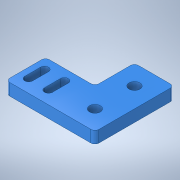
# Autodesk Inventor part: Belt_Clamp
Saved by Autodesk Inventor 2021 (Build 250183000, 183)
## iProperties
Created: 2021-02-02
Part Number: Belt_Clamp
Material: Generic
Document SubType Name: Modeling
Designer: Jorian Brusind
Density: 1 g/cm^3
Appearance: Cyan
Author: Jorian Brusind
Autodesk Inventor part; units mm, degrees
ref_plane "YZ Plane" through (0, 0, 0) normal (1, 0, 0) x (0, 1, 0)
ref_plane "XZ Plane" through (0, 0, 0) normal (0, 1, 0) x (-1, 0, 0)
ref_plane "XY Plane" through (0, 0, 0) normal (0, 0, 1) x (1, 0, 0)
sketch "Sketch1" plane through (0, 0, 0) normal (0, 1, 0) x (-1, 0, 0)
  line L0 (0, 0) -> (45, 0)
  line L1 (45, 0) -> (45, -40)
  line L2 (45, -40) -> (0, -40)
  line L3 (0, -40) -> (0, 0)
  line L4 (45, 0) -> (45, -20)
  line L5 (45, -20) -> (20, -20)
  line L6 (20, -20) -> (20, -40)
  dimension "d0" = 45
  dimension "d1" = 40
  dimension "d13" = 20
  dimension "d14" = 25
  constraints: 14 end point, 3 perpendicular, 2 parallel, 1 horizontal, 1 midpoint, 1 point on line
  measures "d0" distance of L1.end L2.end
  measures "d1" distance of L0.end L1.end
  measures "d13" distance of L0.end L4.end
  measures "d14" distance of L4.end L5.end
extrude "Extrusion3" add sketch "Sketch1" along normal blind 6 contours L0 L1 L5 L6 L2 L3
sketch "Sketch4" plane through (0, 6, 0) normal (0, 1, 0) x (1, 0, 0)
  line L0 (-40, 6.5) -> (-40, 14.5) construction
  line L1 (-38, 6.5) -> (-38, 14.5)
  line L2 (-42, 14.5) -> (-42, 6.5)
  arc A0 (-42, 6.5) -> (-38, 6.5) centre (-40, 6.5) ccw
  arc A1 (-38, 14.5) -> (-42, 14.5) centre (-40, 14.5) ccw
  line L3 (-45, 20) -> (-45, 0) projected
  line L4 (-20, 20) -> (-45, 20) projected
  line L5 (-16.5, 12.5) -> (-2.5, 12.5) construction
  line L6 (-45, 0) -> (0, 0) projected
  point P0 (-40, 10.5)
  dimension "d17" = 4
  dimension "d18" = 4
  dimension "d19" = 3
  dimension "d20" = 5.5
  constraints: 10 end point, 4 point on circle, 4 tangent, 2 centre point, 1 horizontal, 1 midpoint, 1 parallel, 1 vertical
  measures "d17" distance of point (-40, 10.5) L0.end
  measures "d18" diameter of A1
  measures "d19" distance between parallel lines of L3 L2
  measures "d20" distance from line of L4 L0.end
extrude "Extrusion4" cut sketch "Sketch4" against normal through all
sketch "Sketch5" plane through (0, 6, 0) normal (0, 1, 0) x (1, 0, 0)
  circle A0 centre (-10, 10) radius 2.5
  circle A1 centre (-10, 30) radius 2.5
  line L0 (-45, 0) -> (0, 0) projected
  line L1 (0, 0) -> (0, 40) projected
  dimension "d29" = 5
  dimension "d30" = 5
  dimension "d31" = 10
  dimension "d32" = 10
  dimension "d33" = 10
  dimension "d34" = 20
  constraints: 2 centre point
  measures "d29" diameter of A0
  measures "d30" diameter of A1
  measures "d31" distance from line of L0 A0.centre
  measures "d32" distance from line of L1 A0.centre
  measures "d33" distance from line of L1 A1.centre
  measures "d34" distance of A0.centre A1.centre
extrude "Extrusion5" cut sketch "Sketch5" against normal up to next
sketch "Sketch8" plane through (0, 6, 0) normal (0, 1, 0) x (1, 0, 0)
  circle A0 centre (-10, 10) radius 2.5 projected
  circle A1 centre (-10, 10) radius 2.75
  circle A2 centre (-10, 30) radius 2.5 projected
  circle A3 centre (-10, 30) radius 2.75
  point P0 (0, 0)
  dimension "d42" = 5.5
  dimension "d43" = 5.5
  constraints: 2 centre point, 2 coincident
  measures "d42" diameter of A1
  measures "d43" diameter of A3
extrude "Extrusion7" cut sketch "Sketch8" against normal blind 10
fillet "Fillet2" radius 2 5 edges at (0, 3, 0) (0, 3, -40) (-20, 3, -40) (-20, 3, -20) (-20, 0, -30)
fillet "Fillet3" radius 2 2 edges at (-45, 3, -20) (-45, 3, 0)
pattern_linear "Rectangular Pattern1" count 2 spacing 10 along (1, 0, 0) of "Extrusion4"
body "Solid2"
